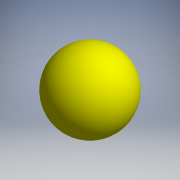
# Autodesk Inventor part: W 619/3-2Z_PART3
Saved by Autodesk Inventor 2017.3 (Build 213256000, 256)
## iProperties
Part Number: W 619/3-2Z_PART3
Material: Generic
Catalog Web Link: www.cadenas.de
Description: -Deep groove ball bearings
Vendor: SKF
Document SubType Name: Modeling
Designer: partserver
Manufacturer: SKF
Mass: 0.000904779 g
Surface Area: 0.0452389 cm^2
Volume: 0.000904779 cm^3
Density: 1 g/cm^3
Appearance: PSOLRGB-192-192-192
Category: PARTsolutions
Company: SKF
Title: W 619/3-2Z_PART3
Author: Cadenas PARTsolutions
Comments: Deep groove ball bearings
PSOL_IDENT_0: {$CADENAS_DATA\23d-libs\skf\bearings_units_and_housings\ball_bearings\deep_groove_ball_bearings\bb1_
PSOL_IDENT_1: 001_101.prj},199 {VTYP=3D},{NB=W 619/3-2Z_PART3},{LINA=W 619/3-2Z_PART3},{NN=BB1_001_101_PART3},{NOP
PSOL_IDENT_2: RJ=TRUE},{DATE=19.12.2019 14:34:47},{GEOMDATE=18.12.2019 13:53:11},{VERSION=},{LINEID=17690},{WBVAR=
PSOL_IDENT_3: },{WBNUMERIC=}  {NB=W 619/3-2Z_PART3},{LINA=W 619/3-2Z_PART3},{KT=DUMMY},{PRODUCTID=1010476193},{DES
PSOL_IDENT_4: IGNATION=W 619/3-2Z},{DD=3.000},{D=8.000},{B=3.000},{C=0.000},{DD1=5.00},{DD2=0.00},{D1=0.00},{D2=7.
PSOL_IDENT_5: 40},{D3=0.000},{D4=0.000},{HH=MIN},{BB=0.000},{FF=0.00},{R0MAX=MIN},{R0=MIN},{R12=0.10},{PITCH=5.90}
PSOL_IDENT_6: ,{DW=1.200},{DDAMIN=3.800},{DDAMAX=4.900},{DDBMIN=MIN},{DDBMAX=MIN},{DBMIN=MIN},{DAMAX=7.500},{BBAMI
PSOL_IDENT_7: N=MIN},{CAMAX=MIN},{RAMAX=0.100},{LOAD1=0.225},{LOAD2=0.072},{LOAD3=0.003},{SPEED1=150000},{SPEED2=7
PSOL_IDENT_8: 5000},{KR=0.025},{F0=7.200},{Z=7},{II=1},{MASS=0.001},{BEARING=W 619/3-2Z},{RING=},{HELP=0.648},{HEL
PSOL_IDENT_9: P2=0.300},{DD1ALG=2.500},{YALG=2.500},{PITCH1=5.900},{DW1=1.200},{YALG1=3.352},{HALG1=0.648},{SH=2.5
PSOL_IDENT_10: 00},{CU=0.360},{DESIGN=dgbbw2z},{HALG=1},{B1=0},{SHIELDHELP=2}
NB: W 619/3-2Z_PART3
NT: Deep groove ball bearings
NBSYN: $DESIGNATION._PART3
LINA: W 619/3-2Z_PART3
CATALOG: SKF
SUPPLIER: SKF
ARTICLENO: W 619/3-2Z_PART3
BOMINFO: W 619/3-2Z_PART3
CREATOR: CADENAS GmbH
Autodesk Inventor part; units mm, degrees
ref_plane "YZ Plane" through (0, 0, 0) normal (1, 0, 0) x (0, 1, 0)
ref_plane "XZ Plane" through (0, 0, 0) normal (0, 1, 0) x (-1, 0, 0)
ref_plane "XY Plane" through (0, 0, 0) normal (0, 0, 1) x (1, 0, 0)
sketch "Sketch_6" plane through (0, 0, 0) normal (0, 0, 1) x (1, 0, 0)
  line L0 (2.1, 2.95) -> (0.9, 2.95)
  arc A0 (2.1, 2.95) -> (0.9, 2.95) centre (1.5, 2.95) ccw
  line L1 (2.1, 2.95) -> (0.9, 2.95)
  dimension "d0" = 360
  constraints: 4 end point, 2 point on circle, 1 centre point
revolve "Revolution1" add sketch "Sketch_6" angle 360 about axis through (2.1, 2.95, 0) along (1, 0, 0)
body "Solid1"
